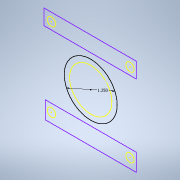
# Autodesk Inventor part: Stepper Spacer Y
Saved by Autodesk Inventor 2020 (Build 240168000, 168)
## iProperties
Created: 2020-03-22
Part Number: Stepper Spacer Y
Material: Generic
Document SubType Name: Modeling
Designer: DasNick
Density: 1 g/cm^3
Appearance: Default
Author: DasNick
Autodesk Inventor part; units mm, degrees
ref_plane "YZ Plane" through (0, 0, 0) normal (1, 0, 0) x (0, 1, 0)
ref_plane "XZ Plane" through (0, 0, 0) normal (0, 1, 0) x (-1, 0, 0)
sketch "Sketch1" plane through (0, 0, 0) normal (0, 0, 1) x (1, 0, 0)
  circle A0 centre (23.57, 23.57) radius 2.5 projected
  circle A1 centre (23.57, -23.57) radius 2.5 projected
  circle A2 centre (-23.57, -23.57) radius 2.5 projected
  circle A3 centre (-23.57, 23.57) radius 2.5 projected
  arc A4 (8.76, 9.1953) -> (9.467, 8.4656) centre (0, 0) ccw projected
  arc A5 (10.897, -6.5227) -> (11.0973, 6.1758) centre (0, 0) ccw projected
  circle A6 centre (0, 0) radius 15.875
  line L0 (-30.405, 29.92) -> (29.92, 29.92)
  line L1 (29.92, 29.92) -> (29.92, 17.22)
  line L2 (29.92, 17.22) -> (-30.405, 17.22)
  line L3 (-30.405, 17.22) -> (-30.405, 29.92)
  line L4 (23.57, 23.57) -> (23.57, -23.57) construction
  line L5 (-23.57, -23.57) -> (-23.57, 23.57) construction
  line L6 (23.57, 0) -> (-23.57, 0) construction
  line L7 (-30.405, -29.92) -> (29.92, -29.92)
  line L8 (29.92, -29.92) -> (29.92, -17.22)
  line L9 (29.92, -17.22) -> (-30.405, -17.22)
  line L10 (-30.405, -17.22) -> (-30.405, -29.92)
  point P0 (0, 0)
  dimension "d0" = 31.75
  dimension "d1" = 6.35
  dimension "d2" = 6.35
  dimension "d3" = 60.325
  dimension "d4" = 6.35
  constraints: 22 end point, 4 symmetric about line, 2 midpoint, 2 parallel, 2 vertical, 1 centre point, 1 coincident, 1 horizontal, 1 perpendicular
  measures "d0" diameter of A6
  measures "d1" distance from line of L2 L4.start
  measures "d2" distance from line of L0 L4.start
  measures "d3" distance between parallel lines of L3 L1
  measures "d4" distance from line of L4.start L1
ref_plane "Work Plane1" through (-28.3245, -28.3245, 68.0874) normal (0, 0, -1) x (0, 1, 0)
extrude "Extrusion1" add sketch "Sketch1" along normal up to surface (68.0874 mm away) contours L0 L1 L2 L3 | L10 L9 L8 L7
body "Solid1"
